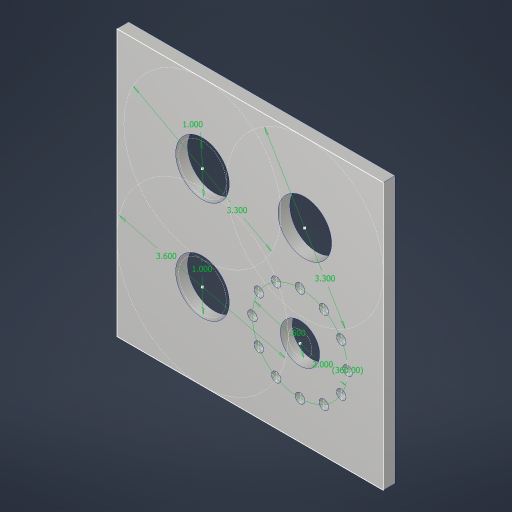
# Autodesk Inventor part: CL4-014
Saved by Autodesk Inventor 2023.4 (Build 274418000, 418)
## iProperties
Created: 2025-02-07
Part Number: CL4-014
Material: Aluminum 6061
Document SubType Name: Modeling
Designer: brand
Density: 2.7 g/cm^3
Appearance: Aluminum - Flat
Author: brand
Autodesk Inventor part; units mm, degrees
ref_plane "YZ Plane" through (0, 0, 0) normal (1, 0, 0) x (0, 1, 0)
ref_plane "XZ Plane" through (0, 0, 0) normal (0, 1, 0) x (-1, 0, 0)
ref_plane "XY Plane" through (0, 0, 0) normal (0, 0, 1) x (1, 0, 0)
sketch "Sketch1" plane through (0, 0, 0) normal (0, 0, 1) x (1, 0, 0)
  circle A0 centre (0, 0) radius 6.35 construction
  circle A1 centre (-52.07, 0) radius 45.72 construction
  circle A2 centre (-52.07, 0) radius 12.7 construction
  circle A3 centre (-52.07, 54.61) radius 41.91 construction
  circle A4 centre (-52.07, 54.61) radius 12.7 construction
  circle A5 centre (2.54, 54.61) radius 41.91 construction
  line L0 (-97.79, 96.52) -> (44.45, 96.52)
  line L1 (44.45, 96.52) -> (44.45, -45.72)
  line L2 (44.45, -45.72) -> (-97.79, -45.72)
  line L3 (-97.79, -45.72) -> (-97.79, 96.52)
  circle A6 centre (0, 0) radius 25.4 construction
  point P0 (25.4, 0)
  point P1 (21.997, 12.7)
  point P2 (12.7, 21.997)
  point P3 (0, 25.4)
  point P4 (-12.7, 21.997)
  point P5 (-21.997, 12.7)
  point P6 (-25.4, 0)
  point P7 (-21.997, -12.7)
  point P8 (-12.7, -21.997)
  point P9 (0, -25.4)
  point P10 (12.7, -21.997)
  point P11 (21.997, -12.7)
  dimension "d15" = 50.8
  dimension "d0" = 12.7
  dimension "d1" = 91.44
  dimension "d2" = 25.4
  dimension "d3" = 83.82
  dimension "d4" = 25.4
  dimension "d5" = 83.82
  dimension "d18" = 360
  constraints: 8 end point, 7 tangent, 6 centre point, 4 coincident, 4 horizontal alignment, 2 parallel, 1 horizontal, 1 perpendicular, 1 vertical alignment, 15 other
  measures "d0" diameter of A0
  measures "d1" diameter of A1
  measures "d2" diameter of A2
  measures "d3" diameter of A3
  measures "d4" diameter of A4
  measures "d5" diameter of A5
extrude "Extrusion1" add sketch "Sketch1" against normal blind 6.35
hole "Hole1" at (-52.07, 0, 0) at (2.54, 54.61, 0) at (-52.07, 54.61, 0) direction (0, 0, -1) diameter 28.575 end through all
hole "Hole2" at (25.4, 0, 0) at (21.997, 12.7, 0) at (12.7, 21.997, 0) at (0, 25.4, 0) at (-12.7, 21.997, 0) at (-21.997, 12.7, 0) at (-25.4, 0, 0) at (-21.997, -12.7, 0) at (-12.7, -21.997, 0) at (0, -25.4, 0) at (12.7, -21.997, 0) at (21.997, -12.7, 0) direction (0, 0, -1) diameter 5.1054 end through all clearance for "Flat Head Machine Screw (82)" size "#10" standard "Ansi Unified Screw Threads"
hole "Hole3" at (0, 0, 0) direction (0, 0, -1) diameter 20.955 end through all
body "Solid1"
